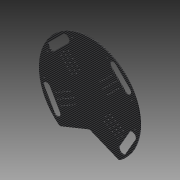
# Autodesk Inventor part: Middle Plate
Saved by Autodesk Inventor 2015 (Build 190159000, 159)
## iProperties
Created: 2016-08-09
Part Number: Middle Plate
Material: Generic
Document SubType Name: Modeling
Designer: James Yelland
Density: 1 g/cm^3
Appearance: Default
Author: James Yelland
Autodesk Inventor part; units mm, degrees
ref_plane "YZ Plane" through (0, 0, 0) normal (1, 0, 0) x (0, 1, 0)
ref_plane "XZ Plane" through (0, 0, 0) normal (0, 1, 0) x (-1, 0, 0)
ref_plane "XY Plane" through (0, 0, 0) normal (0, 0, 1) x (1, 0, 0)
sketch "Sketch1" plane through (0, 0, 0) normal (0, 1, 0) x (-1, 0, 0)
  circle A0 centre (49.6743, 49.6743) radius 1.65
  circle A1 centre (39.8101, 55.1543) radius 1.7
  circle A2 centre (44.3002, 59.6445) radius 1.7
  circle A3 centre (54.1644, 54.1644) radius 1.65
  line L0 (54.1644, 54.1644) -> (58.6899, 58.6899)
  circle A4 centre (59.6445, 44.3002) radius 1.7
  circle A5 centre (55.1543, 39.8101) radius 1.7
  circle A6 centre (45.1841, 45.1841) radius 1.65
  circle A7 centre (35.32, 50.6642) radius 1.7
  circle A8 centre (50.6642, 35.32) radius 1.7
  circle A9 centre (40.694, 40.694) radius 1.65
  circle A10 centre (30.8299, 46.1741) radius 1.7
  circle A11 centre (46.1741, 30.8299) radius 1.7
  circle A12 centre (36.2039, 36.2039) radius 1.65
  circle A13 centre (26.3397, 41.6839) radius 1.7
  circle A14 centre (21.8496, 37.1938) radius 1.7
  circle A15 centre (31.7137, 31.7137) radius 1.65
  circle A16 centre (41.6839, 26.3397) radius 1.7
  circle A17 centre (37.1938, 21.8496) radius 1.7
  circle A18 centre (27.2236, 27.2236) radius 1.65
  circle A19 centre (-49.6743, 49.6743) radius 1.65
  circle A20 centre (-55.1543, 39.8101) radius 1.7
  circle A21 centre (-59.6445, 44.3002) radius 1.7
  circle A22 centre (-54.1644, 54.1644) radius 1.65
  line L1 (-54.1644, 54.1644) -> (-58.6899, 58.6899)
  circle A23 centre (-44.3002, 59.6445) radius 1.7
  circle A24 centre (-39.8101, 55.1543) radius 1.7
  circle A25 centre (-45.1841, 45.1841) radius 1.65
  circle A26 centre (-50.6642, 35.32) radius 1.7
  circle A27 centre (-35.32, 50.6642) radius 1.7
  circle A28 centre (-40.694, 40.694) radius 1.65
  circle A29 centre (-46.1741, 30.8299) radius 1.7
  circle A30 centre (-30.8299, 46.1741) radius 1.7
  circle A31 centre (-36.2039, 36.2039) radius 1.65
  circle A32 centre (-41.6839, 26.3397) radius 1.7
  circle A33 centre (-37.1938, 21.8496) radius 1.7
  circle A34 centre (-31.7137, 31.7137) radius 1.65
  circle A35 centre (-26.3397, 41.6839) radius 1.7
  circle A36 centre (-21.8496, 37.1938) radius 1.7
  circle A37 centre (-27.2236, 27.2236) radius 1.65
  circle A38 centre (-58.0793, -21.0036) radius 1.7
  circle A39 centre (-49.8398, -28.775) radius 1.65
  circle A40 centre (-47.2293, -39.7964) radius 1.7
  circle A41 centre (-52.5801, -17.8286) radius 1.7
  circle A42 centre (-44.3405, -25.6) radius 1.65
  circle A43 centre (-36.2308, -33.4464) radius 1.7
  circle A44 centre (-47.0808, -14.6536) radius 1.7
  circle A45 centre (-41.5816, -11.4786) radius 1.7
  circle A46 centre (-38.8412, -22.425) radius 1.65
  circle A47 centre (-33.342, -19.25) radius 1.65
  circle A48 centre (-30.7316, -30.2714) radius 1.7
  circle A49 centre (-41.7301, -36.6214) radius 1.7
  circle A50 centre (-60.8383, -35.125) radius 1.65
  circle A51 centre (-52.7286, -42.9714) radius 1.7
  circle A52 centre (-58.2279, -46.1464) radius 1.7
  circle A53 centre (-55.339, -31.95) radius 1.65
  circle A54 centre (-63.5786, -24.1786) radius 1.7
  circle A55 centre (-69.0779, -27.3536) radius 1.7
  circle A56 centre (-66.3375, -38.3) radius 1.65
  line L2 (-66.3375, -38.3) -> (-71.8801, -41.5)
  circle A57 centre (47.2293, -39.7964) radius 1.7
  circle A58 centre (49.8398, -28.775) radius 1.65
  circle A59 centre (58.0793, -21.0036) radius 1.7
  circle A60 centre (41.7301, -36.6214) radius 1.7
  circle A61 centre (44.3405, -25.6) radius 1.65
  circle A62 centre (47.0808, -14.6536) radius 1.7
  circle A63 centre (36.2308, -33.4464) radius 1.7
  circle A64 centre (30.7316, -30.2714) radius 1.7
  circle A65 centre (38.8412, -22.425) radius 1.65
  circle A66 centre (33.342, -19.25) radius 1.65
  circle A67 centre (41.5816, -11.4786) radius 1.7
  circle A68 centre (52.5801, -17.8286) radius 1.7
  circle A69 centre (60.8383, -35.125) radius 1.65
  circle A70 centre (63.5786, -24.1786) radius 1.7
  circle A71 centre (69.0779, -27.3536) radius 1.7
  circle A72 centre (55.339, -31.95) radius 1.65
  circle A73 centre (52.7286, -42.9714) radius 1.7
  circle A74 centre (58.2279, -46.1464) radius 1.7
  circle A75 centre (66.3375, -38.3) radius 1.65
  line L3 (66.3375, -38.3) -> (71.8801, -41.5)
  line L4 (-84.8705, -49) -> (-74.3705, -67.1865)
  line L5 (-64.8083, -69.7487) -> (-63.9423, -69.2487)
  line L6 (-61.3801, -59.6865) -> (-82.3801, -23.3135)
  line L7 (-91.9423, -20.7513) -> (-92.8083, -21.2513)
  line L8 (-95.3705, -30.8135) -> (-84.8705, -49)
  arc A76 (-63.9423, -69.2487) -> (-61.3801, -59.6865) centre (-67.4423, -63.1865) ccw
  arc A77 (-74.3705, -67.1865) -> (-64.8083, -69.7487) centre (-68.3083, -63.6865) ccw
  arc A78 (-92.8083, -21.2513) -> (-95.3705, -30.8135) centre (-89.3083, -27.3135) ccw
  arc A79 (-82.3801, -23.3135) -> (-91.9423, -20.7513) centre (-88.4423, -26.8135) ccw
  arc A80 (95.3705, -30.8135) -> (92.8083, -21.2513) centre (89.3083, -27.3135) ccw
  line L9 (92.8083, -21.2513) -> (91.9423, -20.7513)
  line L10 (84.8705, -49) -> (95.3705, -30.8135)
  arc A81 (91.9423, -20.7513) -> (82.3801, -23.3135) centre (88.4423, -26.8135) ccw
  line L11 (74.3705, -67.1865) -> (84.8705, -49)
  arc A82 (64.8083, -69.7487) -> (74.3705, -67.1865) centre (68.3083, -63.6865) ccw
  line L12 (63.9423, -69.2487) -> (64.8083, -69.7487)
  line L13 (82.3801, -23.3135) -> (61.3801, -59.6865)
  arc A83 (61.3801, -59.6865) -> (63.9423, -69.2487) centre (67.4423, -63.1865) ccw
  arc A84 (54.4472, 84.1457) -> (44.5477, 84.1457) centre (49.4975, 79.196) ccw
  line L14 (44.5477, 84.1457) -> (43.8406, 83.4386)
  line L15 (69.2965, 69.2965) -> (54.4472, 84.1457)
  arc A85 (43.8406, 83.4386) -> (43.8406, 73.5391) centre (48.7904, 78.4889) ccw
  line L16 (84.1457, 54.4472) -> (69.2965, 69.2965)
  arc A86 (84.1457, 44.5477) -> (84.1457, 54.4472) centre (79.196, 49.4975) ccw
  line L17 (83.4386, 43.8406) -> (84.1457, 44.5477)
  line L18 (43.8406, 73.5391) -> (73.5391, 43.8406)
  arc A87 (73.5391, 43.8406) -> (83.4386, 43.8406) centre (78.4889, 48.7904) ccw
  arc A88 (-84.1457, 54.4472) -> (-84.1457, 44.5477) centre (-79.196, 49.4975) ccw
  line L19 (-84.1457, 44.5477) -> (-83.4386, 43.8406)
  line L20 (-69.2965, 69.2965) -> (-84.1457, 54.4472)
  arc A89 (-83.4386, 43.8406) -> (-73.5391, 43.8406) centre (-78.4889, 48.7904) ccw
  line L21 (-54.4472, 84.1457) -> (-69.2965, 69.2965)
  arc A90 (-44.5477, 84.1457) -> (-54.4472, 84.1457) centre (-49.4975, 79.196) ccw
  line L22 (-43.8406, 83.4386) -> (-44.5477, 84.1457)
  line L23 (-73.5391, 43.8406) -> (-43.8406, 73.5391)
  arc A91 (-43.8406, 73.5391) -> (-43.8406, 83.4386) centre (-48.7904, 78.4889) ccw
  circle A92 centre (-87.3251, 36.723) radius 1.6
  circle A93 centre (-36.723, 87.3251) radius 1.6
  circle A94 centre (-94.3073, -13.0816) radius 1.6
  circle A95 centre (87.3251, 36.723) radius 1.6
  circle A96 centre (36.723, 87.3251) radius 1.6
  circle A97 centre (94.3073, -13.0816) radius 1.6
  arc A98 (63.9578, -83.273) -> (-63.9578, -83.273) centre (0, 0) ccw
  circle A99 centre (77.9631, 39.7242) radius 1.6
  circle A100 centre (-77.9631, 39.7242) radius 1.6
  line L24 (1.8791, -60.7621) -> (59.0331, -83.9411)
  line L25 (-1.8791, -60.7621) -> (-59.0331, -83.9411)
  arc A101 (59.0331, -83.9411) -> (63.9578, -83.273) centre (60.9122, -79.3076) ccw
  arc A102 (1.8791, -60.7621) -> (-1.8791, -60.7621) centre (0, -65.3955) ccw
  arc A103 (-63.9578, -83.273) -> (-59.0331, -83.9411) centre (-60.9122, -79.3076) ccw
  circle A104 centre (0, 0) radius 75
  point P0 (-78.4889, -38.8909)
  point P1 (-89.0955, -49.4975)
  point P2 (98.8705, -24.7513)
  point P3 (85.8801, -17.2513)
  point P4 (70.8705, -73.2487)
  point P5 (57.8801, -65.7487)
  point P6 (49.4975, 89.0955)
  point P7 (38.8909, 78.4889)
  point P8 (89.0955, 49.4975)
  point P9 (78.4889, 38.8909)
  point P10 (-89.0955, 49.4975)
  point P11 (-78.4889, 38.8909)
  point P12 (-49.4975, 89.0955)
  point P13 (-38.8909, 78.4889)
  point P14 (-61.6441, -85)
  point P15 (61.6441, -85)
  dimension "d27" = 3.2
  dimension "d28" = 3.2
  dimension "d32" = 5
  dimension "d34" = 150
  constraints: 105 centre point, 52 end point, 42 point on circle, 29 point on line, 6 tangent, 2 equal radius, 1 coincident
  measures "d27" diameter of A99
  measures "d28" diameter of A100
  measures "d32" radius of A101
  measures "d34" diameter of A104
extrude "Extrusion1" add sketch "Sketch1" along normal blind 2 contours A2 A104 A23 A22 A21 A55 A56 A52 L25 A103 A98 A101 L24 A74 A75 A71 A4 A3 | A2 A104 A3 A4 A71 A75 A74 L24 A102 L25 A52 A56 A55 A21 A22 A23 | A99 | A100
body "Solid1"
